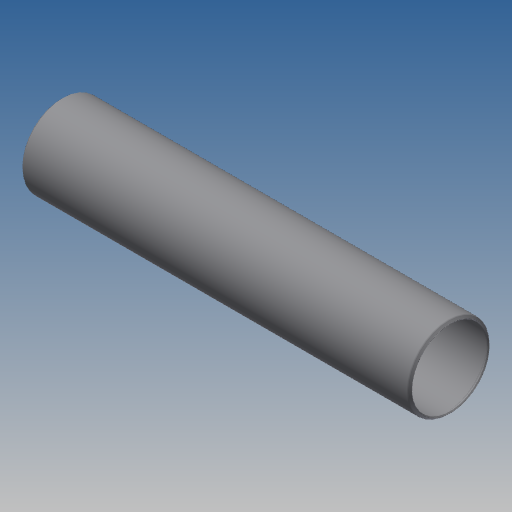
# Autodesk Inventor part: 17R-7.30250C
Saved by Autodesk Inventor 2020 (Build 240168000, 168)
## iProperties
Created: 2020-02-18
Part Number: 17R-7.30250C
Material: Generic
Catalog Web Link: www.cadenas.de
Description: Tube-Original Line - Standard Air Cylinders
Vendor: BIMBA
Document SubType Name: Modeling
Designer: psadmin
Manufacturer: BIMBA
Mass: 13.2812 g
Surface Area: 460.917 cm^2
Volume: 13.2812 cm^3
Density: 1 g/cm^3
Appearance: PSOLRGB-180-180-180
Category: PARTsolutions
Company: BIMBA
PSOL_IDENT_0: {$CADENAS_DATA\23d-libs\bimba\bimba_brand\bimba_imperial\bimba_full_line\original_line_cylinders\sta
PSOL_IDENT_1: ndard_air_cylinders\tube.prj},201 {VTYP=3D},{NB=17R-7.30250C},{LINA=17R-7.30250C},{NN=Tube},{DATE=10
PSOL_IDENT_2: .02.2020 11:56:00},{GEOMDATE=18.02.2011 00:00:00},{VERSION=},{LINEID=80},{WBVAR=MNT,ACTING,NR,L,FOUR
PSOL_IDENT_3: HOLES,SR},{WBNUMERIC=L,FOURHOLES}  {NB=17R-7.30250C},{LINA=17R-7.30250C},{KT=DUMMY},{PN=17R-7.30250C
PSOL_IDENT_4: },{BORE=1.50000000},{BOREPN=17},{MNT=},{MNTALG='' , 'Front Nose' , 'BF' , 'Front Block' , 'BFT' , 'F
PSOL_IDENT_5: ront Trunnion' , 'A' , 'Adjustable Stroke'},{ACTING=R},{ACTINGALG= '' , 'Single Acting' , 'R' , 'Rev
PSOL_IDENT_6: erse/Double Acting' },{NR=},{NRALG= '' , 'Without Non-rotating Rod' , 'NR' , 'With Non-rotating Rod'
PSOL_IDENT_7: },{L=7.3025},{OD=1.5565},{ODN=1.5565},{ODP=1.5565},{ODB=1.5800},{ID=1.5115},{DV=0.00000000},{LV=0.0
PSOL_IDENT_8: 0000000},{LV1=0.00000000},{G=0.0400},{FOURHOLES=0},{AA=0.3750},{BB=0.1250},{SR=C},{SRALG= 'C' , 'Car
PSOL_IDENT_9: bon Steel Rod' , 'SR' , '303 Stainless Steel Rod' , '' , '303 Stainless Steel Rod'}
NN: Tube
NT: Original Line - Standard Air Cylinders
NB: 17R-7.30250C
NBSYN: $PN.
LINA: 17R-7.30250C
BORE: 0
BOREPN: 17
MNT: Front Nose
MNTALG: '' , 'Front Nose' , 'BF' , 'Front Block' , 'BFT' , 'Front Trunnion' , 'A' , 'Adjustable Stroke'
ACTING: Reverse/Double Acting
NR: Without Non-rotating Rod
L: 7.3025
ODN: 1.5565
ODP: 1.5565
ODB: 1.58
ID: 1.5115
DV: 0
LV: 0
LV1: 0
G: 0.04
FOURHOLES: 0
AA: 0.375
BB: 0.125
SR: Carbon Steel Rod
SUPPLIER: BIMBA
ARTICLENO: 17R-7.30250C
BOMINFO: 17R-7.30250C
CREATOR: CADENAS GmbH
Title: 17R-7.30250C
Author: Cadenas PARTsolutions
Comments: Original Line - Standard Air Cylinders
Autodesk Inventor part; units mm, degrees
sketch "Sketch_1" plane through (0, 0, 0) normal (0, 0, 1) x (1, 0, 0)
  line L0 (185.4835, 0) -> (0, 0)
  arc A0 (-0.8826, 18.7343) -> (-0.8826, 18.5547) centre (-0.7928, 18.6445) ccw
  line L1 (-0.8826, 18.5547) -> (-0.508, 18.1801)
  line L2 (-0.508, 18.1801) -> (0, 18.1801)
  line L3 (0, 18.1801) -> (1.016, 19.196)
  line L4 (1.016, 19.196) -> (184.4675, 19.196)
  line L5 (184.4675, 19.196) -> (185.4835, 18.1801)
  line L6 (185.4835, 18.1801) -> (185.9915, 18.1801)
  line L7 (185.9915, 18.1801) -> (186.3661, 18.5547)
  arc A1 (186.3661, 18.5547) -> (186.3661, 18.7343) centre (186.2763, 18.6445) ccw
  line L8 (186.3661, 18.7343) -> (185.6304, 19.47)
  arc A2 (185.6304, 19.47) -> (184.912, 19.7675) centre (184.912, 18.7515) ccw
  line L9 (184.912, 19.7675) -> (0.5715, 19.7675)
  arc A3 (0.5715, 19.7675) -> (-0.1469, 19.47) centre (0.5715, 18.7515) ccw
  line L10 (-0.1469, 19.47) -> (-0.8826, 18.7343)
  constraints: 22 end point, 8 point on circle, 4 centre point
revolve "Revolution1" add sketch "Sketch_1" angle 360 about axis through (185.4835, 0, 0) along (1, 0, 0)
ref_plane "cp1_XY" through (92.7417, 19.7675, 0) normal (1, 0, 0) x (0, 0, -1)
ref_plane "cp1_YZ" through (92.7417, 19.7675, 0) normal (0, 0, -1) x (0, 1, 0)
ref_plane "cp1_ZX" through (92.7417, 19.7675, 0) normal (0, 1, 0) x (1, 0, 0)
ref_plane "cp2_XY" through (92.7417, 0, -19.7675) normal (1, 0, 0) x (0, 0, -1)
ref_plane "cp2_YZ" through (92.7417, 0, -19.7675) normal (0, 0, -1) x (0, 1, 0)
ref_plane "cp2_ZX" through (92.7417, 0, -19.7675) normal (0, 1, 0) x (1, 0, 0)
ref_plane "cp3_XY" through (92.7417, -19.7675, 0) normal (1, 0, 0) x (0, 0, -1)
ref_plane "cp3_YZ" through (92.7417, -19.7675, 0) normal (0, 0, -1) x (0, 1, 0)
ref_plane "cp3_ZX" through (92.7417, -19.7675, 0) normal (0, 1, 0) x (1, 0, 0)
ref_plane "cp4_XY" through (92.7417, 0, 19.7675) normal (1, 0, 0) x (0, 0, -1)
ref_plane "cp4_YZ" through (92.7417, 0, 19.7675) normal (0, 0, -1) x (0, 1, 0)
ref_plane "cp4_ZX" through (92.7417, 0, 19.7675) normal (0, 1, 0) x (1, 0, 0)
ref_plane "tube_front_XY" through (0, 0, 0) normal (1, 0, 0) x (0, 0, -1)
ref_plane "tube_front_YZ" through (0, 0, 0) normal (0, 0, -1) x (0, 1, 0)
ref_plane "tube_front_ZX" through (0, 0, 0) normal (0, 1, 0) x (1, 0, 0)
ref_plane "tube_rear_XY" through (185.4835, 0, 0) normal (1, 0, 0) x (0, 0, -1)
ref_plane "tube_rear_YZ" through (185.4835, 0, 0) normal (0, 0, -1) x (0, 1, 0)
ref_plane "tube_rear_ZX" through (185.4835, 0, 0) normal (0, 1, 0) x (1, 0, 0)
body "Solid1"
